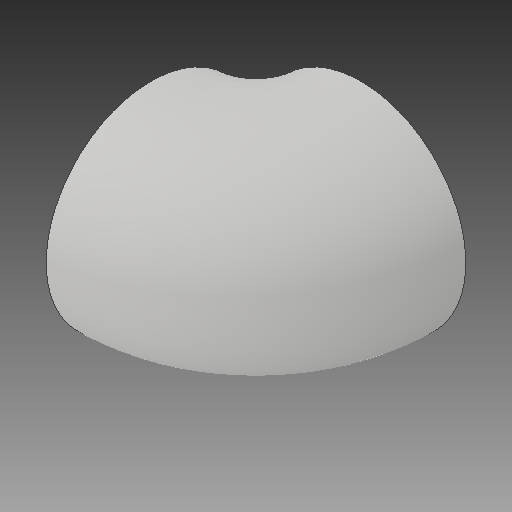
# Autodesk Inventor part: corridor turn
Saved by Autodesk Inventor 2017 (Build 210142000, 142)
## iProperties
Created: 2018-03-04
Part Number: corridor turn
Material: Generic
Document SubType Name: Modeling
Designer: Braxton
Density: 1 g/cm^3
Appearance: Default
Author: Braxton
Autodesk Inventor part; units mm, degrees
ref_plane "YZ Plane" through (0, 0, 0) normal (1, 0, 0) x (0, 1, 0)
ref_plane "XZ Plane" through (0, 0, 0) normal (0, 1, 0) x (-1, 0, 0)
ref_plane "XY Plane" through (0, 0, 0) normal (0, 0, 1) x (1, 0, 0)
sketch "Sketch1" plane through (0, 0, 0) normal (1, 0, 0) x (0, 1, 0)
  line L0 (-84.6667, 50.8) -> (-84.6667, -50.8)
  arc A0 (-110.0667, -57.4059) -> (-110.0667, 57.4059) centre (0, 0) ccw
  arc A1 (84.6667, 50.8) -> (-84.6667, 50.8) centre (0, 0) ccw
  arc A2 (-84.6667, -50.8) -> (84.6667, -50.8) centre (0, 0) ccw
  line L1 (130.9567, -124.1375) -> (-138.9472, -124.1375) construction
  line L2 (-110.0667, -57.4059) -> (-110.0667, 57.4059)
  line L3 (84.6667, 8.9958) -> (84.6667, -8.9958) construction
  arc A3 (84.6667, 8.9958) -> (86.2542, 7.4083) centre (86.2542, 8.9958) ccw
  arc A4 (86.2542, -7.4083) -> (84.6667, -8.9958) centre (86.2542, -8.9958) ccw
  line L4 (84.6667, 0) -> (87.8417, 0) construction
  line L5 (87.8417, 7.4083) -> (86.2542, 7.4083)
  line L6 (87.8417, -7.4083) -> (86.2542, -7.4083)
  line L7 (87.8417, 7.4083) -> (87.8417, -7.4083)
  line L8 (84.6667, -50.8) -> (84.6667, -8.9958)
  line L9 (84.6667, 8.9958) -> (84.6667, 50.8)
  point P0 (84.6667, 0)
  dimension "d1" = 101.6
  dimension "d11" = 25.4
  dimension "d16" = 14.8167
  dimension "d17" = 1.5875
  dimension "d18" = 1.5875
  constraints: 20 end point, 11 point on circle, 5 centre point, 3 symmetric about line, 3 vertical, 2 coincident, 2 tangent, 1 collinear, 1 horizontal, 1 midpoint, 1 other
  measures "d1" distance of L9.end L8.start
  measures "d11" distance between parallel lines of L2 L0
  measures "d16" distance of L5.start L6.start
  measures "d17" distance from line of L8.end L6
  measures "d18" radius of A4
revolve "corridor" add sketch "Sketch1" angle 90 about axis through (0, 130.9567, -124.1375) along (0, 1, 0)
sketch "Sketch4" plane through (0, -110.0667, -57.4059) normal (-1, 0, 0) x (0, 0, 1)
  line L0 (51.0559, 197.9083) -> (57.4059, 197.9083)
  line L1 (64.8142, 197.9083) -> (49.9976, 197.9083)
  line L2 (51.0559, 197.9083) -> (51.0559, 196.6845)
  line L3 (53.3024, 194.7127) -> (57.4059, 194.7127)
  line L4 (57.4059, 194.7127) -> (57.4059, 197.9083) construction
  line L5 (51.0574, 194.7333) -> (54.2316, 197.9076) construction
  arc A0 (54.2323, 194.7127) -> (51.0559, 197.9083) centre (51.0574, 194.7333) ccw construction
  arc A1 (51.0559, 196.6845) -> (53.3024, 194.7127) centre (53.3024, 196.9784) ccw
  line L6 (63.7559, 197.9083) -> (57.4059, 197.9083)
  line L7 (63.7559, 197.9083) -> (63.7559, 196.6845)
  line L8 (61.5093, 194.7127) -> (57.4059, 194.7127)
  line L9 (63.7544, 194.7333) -> (60.5801, 197.9076) construction
  arc A2 (63.7559, 197.9083) -> (60.5795, 194.7127) centre (63.7544, 194.7333) ccw construction
  arc A3 (61.5093, 194.7127) -> (63.7559, 196.6845) centre (61.5093, 196.9784) ccw
  line L10 (64.8142, 197.9083) -> (-66.7316, 197.9083) projected
  line L11 (49.9976, 196.3208) -> (49.9976, 197.9083) projected
  line L12 (-66.7316, 234.2041) -> (-66.7316, 0) construction
  line L13 (-66.7316, 234.2041) -> (-66.7316, 0)
  point P0 (57.4059, 110.0667)
  point P1 (57.4059, 197.9083)
  point P2 (-66.7316, 110.0667)
  dimension "d20" = 6.35
  dimension "d21" = 3.175
  dimension "d22" = 45
  dimension "d23" = 2.2657
  dimension "d24" = 2.2466
  constraints: 22 end point, 10 point on circle, 8 symmetric about line, 5 point on line, 4 centre point, 2 coincident, 2 perpendicular, 1 collinear, 1 horizontal, 1 midpoint, 1 tangent, 1 vertical, 2 other
  measures "d20" distance of L4.end L0.start
  measures "d21" distance of L0.start L5.start
  measures "d22" angle of L0 L5
  measures "d23" radius of A1
  measures "d24" horizontal distance of L3.start L2.end
revolve "light" add sketch "Sketch4" angle 90 about axis through (0, 124.1375, -124.1375) along (0, 1, 0) separate body
equation "\"d17\" = 0.5 * d19"
equation "\"d19\" = 3.175"
body "Solid1"
body "Solid2"
